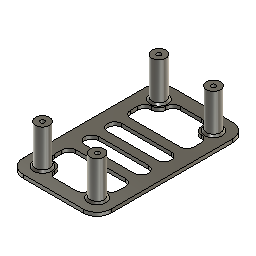
Landing Struts v34 (Autodesk Fusion 360 design; units mm, degrees)
Autodesk Fusion 360 part; units mm, degrees
note: some values were not read from the file. Set by a fixed rule: which sketch regions a step uses.
sketch "Sketch1" plane through (0, 0, 0) normal (0, 0, 1) x (1, 0, 0)
  line L0 (25, 42.5) -> (-25, 42.5)
  line L1 (-25, 42.5) -> (-25, -42.5)
  line L2 (-25, -42.5) -> (25, -42.5)
  line L3 (25, -42.5) -> (25, 42.5)
  line L4 (25, 42.5) -> (-25, -42.5) construction
  line L5 (-25, 42.5) -> (25, -42.5) construction
  line L6 (25, 42.5) -> (46.6506, 55)
  line L7 (25, 42.5) -> (55, 42.5) construction
  line L8 (0, 42.5) -> (0, -42.5)
  line L9 (-25, 0) -> (25, 0)
  line L10 (25, 42.5) -> (23.5, 45.0981)
  line L11 (23.5, 45.0981) -> (45.1506, 57.5981)
  line L12 (45.1506, 57.5981) -> (46.6506, 55)
  line L13 (25, 42.5) -> (26.5, 39.9019)
  line L14 (26.5, 39.9019) -> (48.1506, 52.4019)
  line L15 (23.5, 45.0981) -> (19, 42.5)
  line L16 (26.5, 39.9019) -> (25, 39.0359)
  line L17 (48.1506, 52.4019) -> (46.6506, 55)
  circle A0 centre (46.6506, 55) radius 8.75
  circle A1 centre (46.6506, 55) radius 7.75
  line L18 (46.6506, 55) -> (42.7756, 61.7117)
  line L19 (46.6506, 55) -> (53.3623, 58.875)
  line L20 (46.6506, 55) -> (50.5256, 48.2883)
  circle A2 centre (46.6506, 55) radius 1.5
  line L21 (46.6506, 55) -> (50.9808, 57.5)
  circle A3 centre (50.9808, 57.5) radius 1.1
  circle A4 centre (42.3205, 52.5) radius 1.1
  line L22 (46.6506, 55) -> (44.1506, 59.3301)
  circle A5 centre (44.1506, 59.3301) radius 1.1
  circle A6 centre (49.1506, 50.6699) radius 1.1
  circle A7 centre (-49.1506, 50.6699) radius 1.1
  circle A8 centre (-50.9808, 57.5) radius 1.1
  circle A9 centre (-44.1506, 59.3301) radius 1.1
  circle A10 centre (-46.6506, 55) radius 1.5
  circle A11 centre (-42.3205, 52.5) radius 1.1
  line L23 (-23.5, 45.0981) -> (-45.1506, 57.5981)
  line L24 (-26.5, 39.9019) -> (-48.1506, 52.4019)
  circle A12 centre (-46.6506, 55) radius 8.75
  circle A13 centre (-46.6506, 55) radius 7.75
  line L25 (-26.5, 39.9019) -> (-25, 39.0359)
  line L26 (-23.5, 45.0981) -> (-19, 42.5)
  circle A14 centre (-46.6506, -55) radius 7.75
  circle A15 centre (-44.1506, -59.3301) radius 1.1
  circle A16 centre (-46.6506, -55) radius 1.5
  circle A17 centre (-49.1506, -50.6699) radius 1.1
  circle A18 centre (-42.3205, -52.5) radius 1.1
  circle A19 centre (-50.9808, -57.5) radius 1.1
  line L27 (-26.5, -39.9019) -> (-48.1506, -52.4019)
  line L28 (-23.5, -45.0981) -> (-45.1506, -57.5981)
  line L29 (-23.5, -45.0981) -> (-19, -42.5)
  line L30 (-26.5, -39.9019) -> (-25, -39.0359)
  line L31 (23.5, -45.0981) -> (19, -42.5)
  line L32 (26.5, -39.9019) -> (25, -39.0359)
  line L33 (26.5, -39.9019) -> (48.1506, -52.4019)
  line L34 (23.5, -45.0981) -> (45.1506, -57.5981)
  circle A20 centre (46.6506, -55) radius 8.75
  circle A21 centre (46.6506, -55) radius 7.75
  circle A22 centre (49.1506, -50.6699) radius 1.1
  circle A23 centre (46.6506, -55) radius 1.5
  circle A24 centre (42.3205, -52.5) radius 1.1
  circle A25 centre (44.1506, -59.3301) radius 1.1
  circle A26 centre (50.9808, -57.5) radius 1.1
  circle A27 centre (-46.6506, -55) radius 7.75
  circle A28 centre (-46.6506, -55) radius 8.75
  line L35 (25, 0) -> (25, -42.5)
  line L36 (0, 0) -> (0, -9)
  line L37 (0, -9) -> (0, -10.6)
  line L38 (0, -9) -> (0, -7.4)
  line L39 (0, -9) -> (1, -9)
  line L40 (19, -42.5) -> (25.9282, -46.5)
  line L41 (25, -39.0359) -> (25.0866, -34.0366)
  line L42 (19, -42.5) -> (16, -42.5)
  line L43 (19, -42.5) -> (14.6699, -40)
  line L44 (14.6699, -40) -> (34.8771, -40) construction
  line L45 (25, -39.0359) -> (17.5453, -34.8631)
  line L46 (14.6699, -40) -> (17.5453, -34.8631)
  line L47 (17.5453, -34.8631) -> (25, -21.5453)
  line L48 (25, -42.5) -> (25, -33)
  line L49 (25, -33) -> (15.5, -33)
  circle A29 centre (15.5, -33) radius 2.3
  circle A30 centre (15.5, -33) radius 4
  line L50 (-25, -42.5) -> (-18, -42.5)
  line L51 (-18, -42.5) -> (-18, -27.5)
  line L52 (-18, 42.5) -> (-18, 27.5)
  line L53 (-25, 42.5) -> (-18, 42.5)
  line L54 (18, 42.5) -> (18, 27.5)
  line L55 (18, -42.5) -> (18, -27.5)
  line L56 (18, -30) -> (18, 27.5)
  line L57 (18, 27.5) -> (-18, 27.5)
  line L58 (-18, 27.5) -> (-18, -27.5)
  line L59 (18, -27.5) -> (-18, -27.5)
  circle A31 centre (15.5, -33) radius 1.25
  circle A32 centre (-15.5, -33) radius 1.25
  circle A33 centre (-15.5, -33) radius 2.3
  circle A34 centre (-15.5, -33) radius 4
  circle A35 centre (-15.5, 33) radius 4
  circle A36 centre (-15.5, 33) radius 2.3
  circle A37 centre (-15.5, 33) radius 1.25
  circle A38 centre (15.5, 33) radius 1.25
  circle A39 centre (15.5, 33) radius 2.3
  circle A40 centre (15.5, 33) radius 4
  line L60 (18, 27.5) -> (18, 15.5)
  line L61 (18, 15.5) -> (-18, 15.5)
  line L62 (18, 15.5) -> (18, 10.5)
  line L63 (18, 10.5) -> (-18, 10.5)
  line L64 (18, -10.5) -> (-18, -10.5)
  line L65 (18, -15.5) -> (-18, -15.5)
  line L66 (0, 0) -> (0, 2.5)
  line L67 (0, 2.5) -> (-18, 2.5)
  line L68 (0, 2.5) -> (18, 2.5)
  line L69 (0, -2.5) -> (18, -2.5)
  line L70 (0, -2.5) -> (-18, -2.5)
  line L71 (0, 27.5) -> (10, 27.5)
  line L72 (10, 27.5) -> (10, 42.5)
  line L73 (-10, 27.5) -> (-10, 42.5)
  line L74 (10, 42.5) -> (10, 35.5)
  line L75 (10, 35.5) -> (-10, 35.5)
  line L76 (10, -35.5) -> (-10, -35.5)
  line L77 (-10, -27.5) -> (-10, -42.5)
  line L78 (10, -27.5) -> (10, -42.5)
  point P0 (-46.6506, -55)
  dimension "d1" = 50
  dimension "d2" = 85
  dimension "d4" = 25
  dimension "d5" = 30
  dimension "d6" = 3
  dimension "d7" = 25
  dimension "d8" = 17.5
  dimension "d9" = 15.5
  dimension "d10" = 3
  dimension "d11" = 5
  dimension "d12" = 2.2
  dimension "d13" = 5
  dimension "d14" = 2.2
  dimension "d23" = 9
  dimension "d24" = 1.6
  dimension "d25" = 1.6
  dimension "d51" = 8
  dimension "d76" = 5
  dimension "d77" = 3
  dimension "d88" = 5
  dimension "d130" = 180
  dimension "d131" = 9.5
  dimension "d132" = 9.5
  dimension "d133" = 4.6
  dimension "d134" = 8
  dimension "d141" = 7
  dimension "d142" = 15
  dimension "d170" = 2.5
  dimension "d180" = 12
  dimension "d181" = 5
  dimension "d182" = 2.5
  dimension "d186" = 10
  dimension "d187" = 7
  constraint horizontal L0
  constraint perpendicular L0 L1
  constraint parallel L0 L2
  constraint parallel L1 L3
  constraint coincident L4 L36.start
  constraint coincident L5 L36.start
  constraint coincident L36.start L66.start
  constraint horizontal L7
  constraint midpoint L0 L8.start
  constraint midpoint L2 L8.end
  constraint midpoint L1 L9.start
  constraint midpoint L3 L9.end
  constraint perpendicular L6 L10
  constraint perpendicular L10 L11
  constraint symmetric L0.start L6 L3.end
  constraint symmetric L6 L10.end L13.end
  constraint symmetric L6 L11.end L14.end
  constraint coincident L0 L15.end
  constraint perpendicular L10 L15
  constraint coincident L3 L16.end
  constraint perpendicular L13 L16
  constraint symmetric L12.end L6 L17.end
  constraint coincident L6.end L12.end
  constraint concentric A0 A1
  constraint coincident A1 L18.end
  constraint parallel L12 L18
  constraint coincident A1 L19.end
  constraint perpendicular L12 L19
  constraint coincident A1 L20.end
  constraint perpendicular L19 L20
  constraint perpendicular L20 L21
  constraint coincident L21.end A3.centre
  constraint symmetric L18 A3 A4
  constraint parallel L18 L22
  constraint coincident L22.end A5.centre
  constraint symmetric L6 A5 A6
  constraint symmetric L8 L10.end L23.start
  constraint symmetric L8 L11.end L23.end
  constraint symmetric L8 L13.end L24.start
  constraint symmetric L8 L14.end L24.end
  constraint symmetric L8 L15.end L26.end
  constraint symmetric L8 L16.end L25.end
  constraint symmetric L8 A0 A12
  constraint symmetric L8 A1 A13
  constraint symmetric L8 A2 A10
  constraint symmetric L8 A3 A8
  constraint symmetric L8 A4 A11
  constraint symmetric L8 A5 A9
  constraint symmetric L8 A6 A7
  constraint symmetric L9 L10.end L31.start
  constraint symmetric L9 L11.end L34.end
  constraint symmetric L9 L13.end L32.start
  constraint symmetric L9 L14.end L33.end
  constraint symmetric L9 L15.end L31.end
  constraint symmetric L9 L16.end L32.end
  constraint symmetric L9 A0 A20
  constraint symmetric L9 A1 A21
  constraint symmetric L9 A2 A23
  constraint symmetric L9 A3 A26
  constraint symmetric L9 A4 A24
  constraint symmetric L9 A5 A25
  constraint symmetric L9 A6 A22
  constraint symmetric L9 A7 A17
  constraint symmetric L9 A8 A19
  constraint symmetric L9 A9 A15
  constraint symmetric L9 A10 A16
  constraint symmetric L9 A11 A18
  constraint symmetric L9 L23.start L28.start
  constraint symmetric L9 L23.end L28.end
  constraint symmetric L9 L24.start L27.start
  constraint symmetric L9 L24.end L27.end
  constraint symmetric L9 A10.centre P0
  constraint symmetric L9 A13 A14
  constraint symmetric L9 L25.end L30.end
  constraint symmetric L9 L26.end L29.end
  constraint symmetric L9 A13 A27
  constraint symmetric L9 A12 A28
  constraint perpendicular L9 L36
  constraint parallel L8 L37
  constraint parallel L36 L38
  constraint perpendicular L38 L39
  constraint parallel L34 L40
  constraint parallel L2 L42
  constraint parallel L31 L43
  constraint horizontal L44
  constraint perpendicular L45 L46
  constraint coincident L35 L47.end
  constraint perpendicular L2 L48
  constraint perpendicular L48 L49
  constraint coincident L49.end A29.centre
  constraint concentric A29 A30
  constraint perpendicular L1 L50
  constraint perpendicular L50 L51
  constraint symmetric L1.end L9 L0.end
  constraint symmetric L9 L50.end L52.start
  constraint symmetric L9 L51.end L52.end
  constraint symmetric L8 L50.end L55.start
  constraint symmetric L8 L51.end L55.end
  constraint symmetric L8 L52.start L54.start
  constraint symmetric L8 L52.end L54.end
  constraint vertical L56
  constraint horizontal L57
  constraint vertical L58
  constraint symmetric L9 L54.end L55.end
  constraint symmetric L9 L52.end L51.end
  constraint concentric A29 A31
  constraint symmetric L8 A29 A33
  constraint symmetric L8 A30 A34
  constraint symmetric L8 A31 A32
  constraint symmetric L9 A29 A39
  constraint symmetric L9 A30 A40
  constraint symmetric L9 A31 A38
  constraint symmetric L9 A32 A37
  constraint symmetric L9 A33 A36
  constraint symmetric L9 A34 A35
  constraint perpendicular L57 L60
  constraint coincident L58 L61.end
  constraint perpendicular L58 L61
  constraint coincident L56 L62.end
  constraint coincident L58 L63.end
  constraint perpendicular L58 L63
  constraint symmetric L9 L60.end L65.start
  constraint symmetric L9 L61.end L65.end
  constraint symmetric L9 L62.end L64.start
  constraint symmetric L9 L63.end L64.end
  constraint parallel L8 L66
  constraint coincident L58 L67.end
  constraint perpendicular L58 L67
  constraint symmetric L8 L66.end L67.start
  constraint symmetric L8 L67.end L68.end
  constraint symmetric L9 L66.end L69.start
  constraint symmetric L9 L67.end L70.end
  constraint symmetric L9 L68.end L69.end
  constraint midpoint L57 L71.start
  constraint coincident L57 L71.end
  constraint coincident L0 L72.end
  constraint perpendicular L0 L72
  constraint symmetric L8 L71.end L73.start
  constraint symmetric L8 L72.end L73.end
  constraint perpendicular L0 L74
  constraint coincident L73 L75.end
  constraint perpendicular L73 L75
  constraint symmetric L9 L71.end L78.start
  constraint symmetric L9 L72.end L78.end
  constraint symmetric L9 L73.start L77.start
  constraint symmetric L9 L73.end L77.end
  constraint symmetric L9 L74.end L76.start
  constraint symmetric L9 L75.end L76.end
  measures "d1" distance of L1.end L2.end
  measures "d2" distance of L0.end L1.end
  measures "d4" distance of L0.start L6.end
  measures "d5" angle of L6 L7
  measures "d6" distance of L0.start L10.end
  measures "d7" distance of L10.end L11.end
  measures "d8" diameter of A0
  measures "d9" diameter of A1
  measures "d10" diameter of A2
  measures "d11" distance of L6.end L21.end
  measures "d12" diameter of A3
  measures "d13" distance of L6.end L22.end
  measures "d14" diameter of A5
  measures "d23" distance of L36.start L36.end
  measures "d24" distance of L36.end L37.end
  measures "d25" distance of L36.end L38.end
  measures "d51" distance of L31.end L40.end
  measures "d76" distance of L32.end L41.end
  measures "d77" distance of L31.end L42.end
  measures "d88" distance of L31.end L43.end
  measures "d130" angle of L46 L47
  measures "d131" distance of L2.end L48.end
  measures "d132" distance of L48.end L49.end
  measures "d133" diameter of A29
  measures "d134" diameter of A30
  measures "d141" distance of L1.end L50.end
  measures "d142" distance of L50.end L51.end
  measures "d170" diameter of A31
  measures "d180" distance of L54.end L60.end
  measures "d181" distance of L60.end L62.end
  measures "d182" distance of L36.start L66.end
  measures "d186" distance of L71.start L71.end
  measures "d187" distance of L72.end L74.end
extrude "Extrude1" add sketch "Sketch1" along normal blind 2 contours L3 L9 L35 L47 A30 L55 L56 | L3 L35 L47 L49 A30 | L8 L9 L36 L56 L69 | L8 L9 L56 L66 L68 | L3 L35 L45 L48 L49 A30 | L47 L49 A30 | L47 L49 A30 L55 L56 | L8 L36 L37 L38 L56 L64 L69 | L2 L3 L35 L43 L45 L48 A30 L55 | L45 L47 L49 A30 L55 | L47 L49 L55 | L46 L47 A30 L55 L56 | L2 L42 L43 L46 A30 L55 L56 L59 L78 | L8 L37 L56 L64 L65 | L45 A30 L55 | L45 L47 L55 | L43 L46 A30 L55 | L45 L46 A30 L55 | L8 L56 L59 L65 | L2 L42 L43 L55 | L8 L59 L76 L78 | L2 L8 L76 L78
extrude "Extrude3" add sketch "Sketch1" along normal blind 24 contours L47 L49 A30 | L47 L49 A30 L55 L56 | L45 L47 L49 A30 L55 | L47 L49 L55 | L46 L47 A30 L55 L56 | L45 A30 L55 | L45 L47 L55 | L45 L46 A30 L55 | A29
mirror "Mirror3" about plane through (0, -27.5, 0) normal (-1, 0, 0) of bodies 1 merged
extrude "Extrude6" cut sketch "Sketch1" along normal blind 12 contours L8 L36 L37 L38 L56 L64 L69 | L8 L56 L63 L68 | L8 L56 L57 L60 L61 L71 | L8 L58 L63 L67 | L8 L36 L37 L38 L58 L64 L70 | L8 L56 L61 L62 L63 | L8 L57 L58 L61 | L8 L56 L59 L65 | L8 L58 L61 L63 | L8 L58 L59 L65
fillet "Fillet4" radius 8 2 edges at (25, -42.5, 1) (-25, -42.5, 1)
mirror "Mirror5" about plane through (18, 0, 0) normal (0, 1, 0) of bodies 1 merged
fillet "Fillet8" radius 4 4 edges at (18, 27.5, 1) (-18, 27.5, 1) (18, -27.5, 1) (-18, -27.5, 1)
fillet "Fillet9" radius 4 12 edges at (-18, -15.5, 1) (-18, -10.5, 1) (-18, -2.5, 1) (-18, 2.5, 1) (18, 2.5, 1) (18, -2.5, 1) (18, -10.5, 1) (18, -15.5, 1) (18, 10.5, 1) (-18, 10.5, 1) (-18, 15.5, 1) (18, 15.5, 1)
chamfer "Chamfer46" distance 1 angle 45 4 edges at (11.7707, 31.5535, 2) (-11.7707, 31.5535, 2) (11.7707, -31.5535, 2) (-11.7707, -31.5535, 2)
extrude "Extrude9" cut sketch "Sketch1" along normal blind 7 contours L8 L57 L71 L72 L75 | L8 L57 L73 L75 | L8 L59 L76 L78 | L8 L59 L76 L77
fillet "Fillet10" radius 4 4 edges at (-10, -35.5, 1) (10, -35.5, 1) (10, 35.5, 1) (-10, 35.5, 1)
fillet "Fillet11" radius 4 4 edges at (-10, 27.5, 1) (10, 27.5, 1) (-10, -27.5, 1) (10, -27.5, 1)
